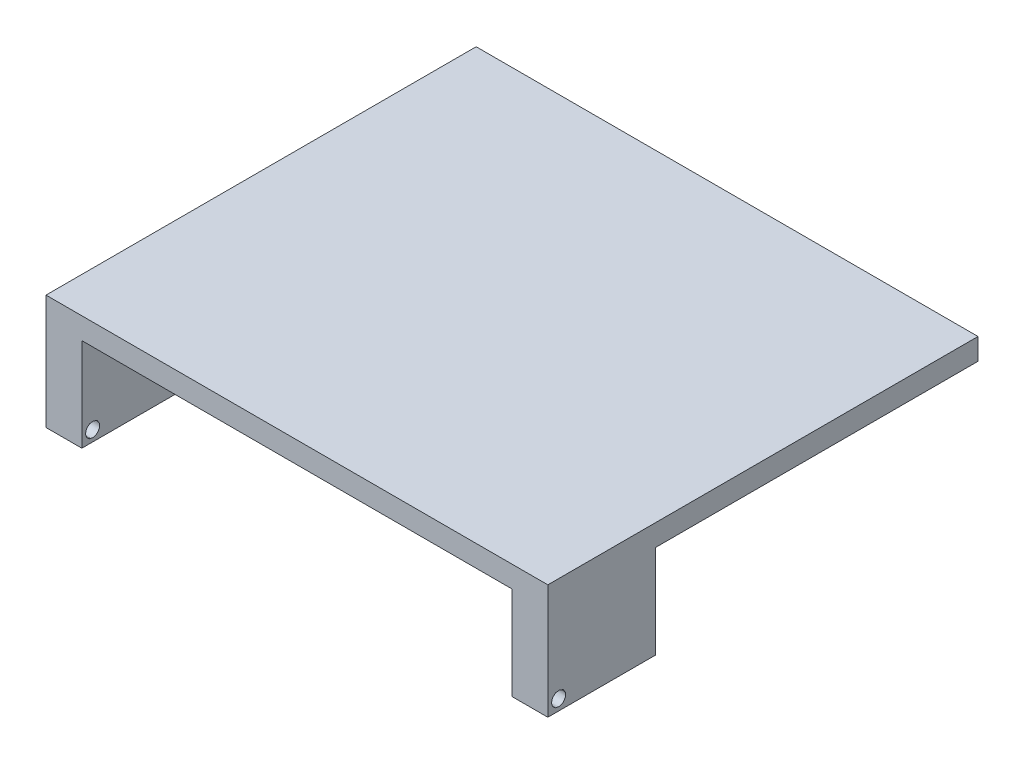
# Autodesk Inventor part: base_3
Saved by Autodesk Inventor 2019 (Build 230136000, 136)
## iProperties
Created: 2020-03-13
Part Number: base_3
Material: Generic
Document SubType Name: Modeling
Designer: Pulag
Density: 1 g/cm^3
Appearance: Default
Author: Pulag
Autodesk Inventor part; units mm, degrees
ref_plane "YZ Plane" through (0, 0, 0) normal (1, 0, 0) x (0, 1, 0)
ref_plane "Work Plane1" through (-35, 0, -35) normal (0, 1, 0) x (1, 0, 0)
ref_plane "Work Plane2" through (-23.7602, 13, -55.0885) normal (0, -1, 0) x (1, 0, 0)
sketch "Sketch1" plane through (-35, 0, -35) normal (0, 1, 0) x (1, 0, 0)
  line L0 (-4, 96.5) -> (-2.5, 96.5) projected
  line L1 (-2.5, 96.5) -> (-2.5, 43.5) projected
  line L2 (-2.5, 43.5) -> (-4, 43.5) projected
  line L3 (-4, 43.5) -> (-4, 96.5) projected
  line L4 (31, 43.5) -> (31, 96.5) projected
  line L5 (31, 96.5) -> (32.5, 96.5) projected
  line L6 (32.5, 96.5) -> (32.5, 43.5) projected
  line L7 (32.5, 43.5) -> (31, 43.5) projected
  line L8 (4, 96.5) -> (4, 43.5) projected
  line L9 (4, 43.5) -> (2.5, 43.5) projected
  line L10 (2.5, 43.5) -> (2.5, 96.5) projected
  line L11 (2.5, 96.5) -> (4, 96.5) projected
  line L12 (-31, 43.5) -> (-32.5, 43.5) projected
  line L13 (-32.5, 43.5) -> (-32.5, 96.5) projected
  line L14 (-32.5, 96.5) -> (-31, 96.5) projected
  line L15 (-31, 96.5) -> (-31, 43.5) projected
  circle A0 centre (0, 0) radius 8.5 projected
  line L16 (-35, -20) -> (-30, -20) projected
  line L17 (-30, -20) -> (-30, -35) projected
  line L18 (-30, -35) -> (30.0078, -35) projected
  line L19 (30.0078, -35) -> (30.0078, -20) projected
  line L20 (30.0078, -20) -> (35, -20) projected
  line L21 (35, -20) -> (35, 105) projected
  line L22 (35, 105) -> (-35, 105) projected
  line L23 (-35, 105) -> (-35, -20) projected
  line L24 (-35, -35) -> (35, -35)
  line L25 (35, -35) -> (35, 25)
  line L26 (35, 25) -> (-35, 25)
  line L27 (-35, 25) -> (-35, -35)
  line L28 (-4, 96.5) -> (-2.5, 96.5)
  line L29 (-2.5, 96.5) -> (-2.5, 43.5)
  line L30 (-2.5, 43.5) -> (-4, 43.5)
  line L31 (-4, 43.5) -> (-4, 96.5)
  line L32 (31, 43.5) -> (31, 96.5)
  line L33 (31, 96.5) -> (32.5, 96.5)
  line L34 (32.5, 96.5) -> (32.5, 43.5)
  line L35 (32.5, 43.5) -> (31, 43.5)
  line L36 (4, 96.5) -> (4, 43.5)
  line L37 (4, 43.5) -> (2.5, 43.5)
  line L38 (2.5, 43.5) -> (2.5, 96.5)
  line L39 (2.5, 96.5) -> (4, 96.5)
  line L40 (-31, 43.5) -> (-32.5, 43.5)
  line L41 (-32.5, 43.5) -> (-32.5, 96.5)
  line L42 (-32.5, 96.5) -> (-31, 96.5)
  line L43 (-31, 96.5) -> (-31, 43.5)
  circle A1 centre (0, 0) radius 8.5
  line L44 (-35, -20) -> (-30, -20)
  line L45 (-30, -20) -> (-30, -35)
  line L46 (-30, -35) -> (30.0078, -35)
  line L47 (30.0078, -35) -> (30.0078, -20)
  line L48 (30.0078, -20) -> (35, -20)
  line L49 (35, -20) -> (35, 105)
  line L50 (35, 105) -> (-35, 105)
  line L51 (-35, 105) -> (-35, -20)
  line L52 (-35, -35) -> (35, -35)
  line L53 (35, -35) -> (35, 25)
  line L54 (35, 25) -> (-35, 25)
  line L55 (-35, 25) -> (-35, -35)
  point P0 (35, -35)
  point P1 (35, -35)
  dimension "d0" = 60
  dimension "d3" = 60
  constraints: 64 end point, 4 parallel, 4 point on line, 2 horizontal, 2 perpendicular, 1 centre point
  measures "d0" distance of L25.end L24.end
  measures "d3" distance of L53.end L52.end
extrude "Extrusion1" add sketch "Sketch1" along normal up to surface (13 mm away) contours A0 | L23 L26 L21 L20 L19 L18 L17 L16 | L16 L17 L24 L27 | L19 L20 L25 L24
sketch "Sketch2" plane through (-35, 0, -35) normal (0, 1, 0) x (1, 0, 0)
  line L0 (-4, 96.5) -> (-2.5, 96.5)
  line L1 (-2.5, 96.5) -> (-2.5, 43.5)
  line L2 (-2.5, 43.5) -> (-4, 43.5)
  line L3 (-4, 43.5) -> (-4, 96.5)
  line L4 (31, 43.5) -> (31, 96.5)
  line L5 (31, 96.5) -> (32.5, 96.5)
  line L6 (32.5, 96.5) -> (32.5, 43.5)
  line L7 (32.5, 43.5) -> (31, 43.5)
  line L8 (4, 96.5) -> (4, 43.5)
  line L9 (4, 43.5) -> (2.5, 43.5)
  line L10 (2.5, 43.5) -> (2.5, 96.5)
  line L11 (2.5, 96.5) -> (4, 96.5)
  line L12 (-31, 43.5) -> (-32.5, 43.5)
  line L13 (-32.5, 43.5) -> (-32.5, 96.5)
  line L14 (-32.5, 96.5) -> (-31, 96.5)
  line L15 (-31, 96.5) -> (-31, 43.5)
  circle A0 centre (0, 0) radius 8.5
  line L16 (-35, -20) -> (-30, -20)
  line L17 (-30, -20) -> (-30, -35)
  line L18 (-30, -35) -> (30.0078, -35)
  line L19 (30.0078, -35) -> (30.0078, -20)
  line L20 (30.0078, -20) -> (35, -20)
  line L21 (35, -20) -> (35, 105)
  line L22 (35, 105) -> (-35, 105)
  line L23 (-35, 105) -> (-35, -20)
  line L24 (-35, -35) -> (35, -35)
  line L25 (35, -35) -> (35, 25)
  line L26 (35, 25) -> (-35, 25)
  line L27 (-35, 25) -> (-35, -35)
  line L28 (-4, 96.5) -> (-2.5, 96.5)
  line L29 (-2.5, 96.5) -> (-2.5, 43.5)
  line L30 (-2.5, 43.5) -> (-4, 43.5)
  line L31 (-4, 43.5) -> (-4, 96.5)
  line L32 (31, 43.5) -> (31, 96.5)
  line L33 (31, 96.5) -> (32.5, 96.5)
  line L34 (32.5, 96.5) -> (32.5, 43.5)
  line L35 (32.5, 43.5) -> (31, 43.5)
  line L36 (4, 96.5) -> (4, 43.5)
  line L37 (4, 43.5) -> (2.5, 43.5)
  line L38 (2.5, 43.5) -> (2.5, 96.5)
  line L39 (2.5, 96.5) -> (4, 96.5)
  line L40 (-31, 43.5) -> (-32.5, 43.5)
  line L41 (-32.5, 43.5) -> (-32.5, 96.5)
  line L42 (-32.5, 96.5) -> (-31, 96.5)
  line L43 (-31, 96.5) -> (-31, 43.5)
  circle A1 centre (0, 0) radius 8.5
  line L44 (-35, -20) -> (-30, -20)
  line L45 (-30, -20) -> (-30, -35)
  line L46 (-30, -35) -> (30.0078, -35)
  line L47 (30.0078, -35) -> (30.0078, -20)
  line L48 (30.0078, -20) -> (35, -20)
  line L49 (35, -20) -> (35, 105)
  line L50 (35, 105) -> (-35, 105)
  line L51 (-35, 105) -> (-35, -20)
  line L52 (-35, -35) -> (35, -35)
  line L53 (35, -35) -> (35, 25)
  line L54 (35, 25) -> (-35, 25)
  line L55 (-35, 25) -> (-35, -35)
  point P0 (35, -35)
  point P1 (35, -35)
  point P2 (35, -35)
  dimension "d4" = 60
  dimension "d5" = 60
  constraints: 112 end point, 4 parallel, 4 point on line, 2 centre point, 2 horizontal, 2 perpendicular
  measures "d4" distance of L25.end L24.end
  measures "d5" distance of L53.end L52.end
extrude "Extrusion2" cut sketch "Sketch2" against normal blind 3 from surface at 13 contours A0 | L23 L26 L21 L20 L19 L18 L17 L16 | L16 L17 L24 L27 | L19 L20 L25 L24 keep common part
sketch "Sketch3" plane through (-70, 10, 0) normal (0, -1, 0) x (1, 0, 0)
  line L0 (5, 0) -> (5, -15) projected
  line L1 (5, -15) -> (0, -15) projected
  line L2 (0, 0) -> (0, -60) projected
  line L3 (70, 0) -> (0, 0) projected
  line L4 (0, 0) -> (0, -60) projected
  line L5 (0, -60) -> (70, -60) projected
  line L6 (70, -60) -> (70, 0) projected
  line L7 (65.0078, -15) -> (65.0078, 0) projected
  line L8 (70, -15) -> (65.0078, -15) projected
  line L9 (70, -60) -> (70, 0) projected
  line L10 (0, -15) -> (5, -15)
  line L11 (5, -15) -> (5, 0)
  line L12 (5, 0) -> (0, 0)
  line L13 (0, 0) -> (0, -15)
  line L14 (65.0078, 0) -> (70, 0)
  line L15 (70, 0) -> (70, -15)
  line L16 (70, -15) -> (65.0078, -15)
  line L17 (65.0078, -15) -> (65.0078, 0)
  constraints: 16 end point, 4 parallel, 2 horizontal, 2 perpendicular
ref_plane "Work Plane3" through (-70.7285, -3, -140.3642) normal (0, -1, 0) x (1, 0, 0)
extrude "Extrusion3" add sketch "Sketch3" along normal up to surface (13 mm away) contours L0 L1 L2 L3 | L3 L6 L8 L7
sketch "Sketch4" plane through (-70, 13, -60) normal (-1, 0, 0) x (0, 0, 1)
  line L0 (45, -16) -> (60, -16) projected
  line L1 (60, -13) -> (64.2426, -13) construction
  circle A0 centre (58.5, -14.5) radius 1
  dimension "d11" = 2
  constraints: 2 end point, 1 centre point, 1 horizontal
  measures "d11" diameter of A0
extrude "Extrusion4" cut sketch "Sketch4" against normal up to surface (70 mm away)
body "Solid1"
